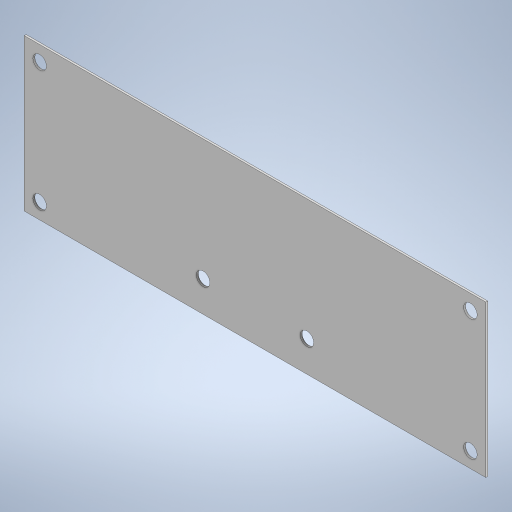
# Autodesk Inventor part: magnet_test_print_v02
Saved by Autodesk Inventor 2023 (Build 270158000, 158)
## iProperties
Created: 2021-04-13
Part Number: magnet_test_print_v02
Material: Generic
Document SubType Name: Modeling
Designer: KAMPFF-LAB-BEHAVIOR
Density: 1 g/cm^3
Appearance: Default
Author: KAMPFF-LAB-BEHAVIOR
Autodesk Inventor part; units mm, degrees
ref_plane "YZ Plane" through (0, 0, 0) normal (1, 0, 0) x (0, 1, 0)
ref_plane "XZ Plane" through (0, 0, 0) normal (0, 1, 0) x (-1, 0, 0)
ref_plane "XY Plane" through (0, 0, 0) normal (0, 0, 1) x (1, 0, 0)
sketch "Sketch66" plane through (0, 0, 0) normal (0, 0, 1) x (1, 0, 0)
  line L0 (-120, -39.5) -> (120, -39.5)
  line L1 (120, -39.5) -> (120, 39.5)
  line L2 (120, 39.5) -> (-120, 39.5)
  line L3 (-120, 39.5) -> (-120, -39.5)
  line L4 (-120, -39.5) -> (120, 39.5) construction
  line L5 (120, -39.5) -> (-120, 39.5) construction
  point P0 (0, 0)
  dimension "d179" = 240
  dimension "d180" = 79
  constraints: 12 end point, 2 midpoint, 2 parallel, 1 horizontal, 1 perpendicular
  measures "d179" distance of L2.end L1.end
  measures "d180" distance of L1.end L0.end
extrude "Extrusion45" add sketch "Sketch66" along normal blind 1
sketch "Sketch68" plane through (0, 0, 1) normal (0, 0, 1) x (1, 0, 0)
  circle A0 centre (-112, 31.5) radius 3.5
  circle A1 centre (-112, -31.5) radius 3.5
  circle A2 centre (112, 31.5) radius 3.5
  circle A3 centre (112, -31.5) radius 3.5
  point P0 (0, 0)
  dimension "d186" = 7
  dimension "d187" = 7
  dimension "d188" = 7
  dimension "d189" = 7
  constraints: 4 centre point
  measures "d186" diameter of A0
  measures "d187" diameter of A1
  measures "d188" diameter of A2
  measures "d189" diameter of A3
extrude "Extrusion47" cut sketch "Sketch68" against normal through all
sketch "Sketch69" plane through (0, 0, 1) normal (0, 0, 1) x (1, 0, 0)
  circle A0 centre (-27, -23.5) radius 3.5
  circle A1 centre (27, -23.5) radius 3.5
  point P0 (0, 0)
  dimension "d192" = 7
  dimension "d193" = 7
  constraints: 2 centre point
  measures "d192" diameter of A0
  measures "d193" diameter of A1
extrude "Extrusion48" cut sketch "Sketch69" against normal through all
equation "\"d187\" = d186"
equation "\"d188\" = d186"
equation "\"d189\" = d186"
equation "\"d192\" = d186"
equation "\"d193\" = d186"
body "Solid10"
